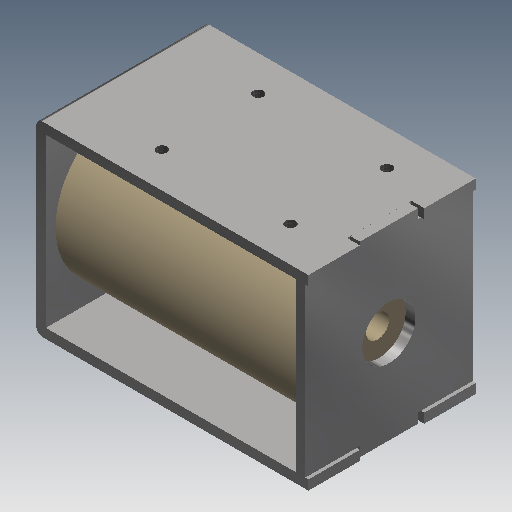
# Autodesk Inventor part: JF_0837B_Linear solenoid Pull 15N 12v1A Frame
Saved by Autodesk Inventor 2018.3 (Build 223284000, 284)
## iProperties
Manager: GURSKY
Company: ltd "MRF-ENGINEERING"
Created: 2017-09-28
Part Number: JF_0837B_Linear solenoid Pull 15N 12v1A Frame
Project: 1706
Checked By: Гурский
Engr Approved By: ---
Material: Сталь нержавеющая, 440C
Catalog Web Link: http://mrfengineering.com.ua/
Vendor: ltd "MRF-ENGINEERING"
Document SubType Name: Листовой металл
Designer: Макс
Engineer: TIHONOV
Authority: GURSKY
Stock Number: 1706
Density: 7.75 g/cm^3
Sheet Metal Rule: Default_mm
Appearance: С умеренной полировкой
Заготовка: ЛИСТ ГОРЯЧЕКАТАННЫЙ 4,0х1500х6000
Материал: Ст. 3СП/ПС
Title: ---
Subject: Filling mashine
Author: Макс
Autodesk Inventor part; units mm, degrees
ref_plane "YZ Plane" through (0, 0, 0) normal (1, 0, 0) x (0, 1, 0)
ref_plane "XZ Plane" through (0, 0, 0) normal (0, 1, 0) x (-1, 0, 0)
ref_plane "XY Plane" through (0, 0, 0) normal (0, 0, 1) x (1, 0, 0)
sketch "Эскиз2" plane through (0, 0, 0) normal (0, 0, 1) x (1, 0, 0)
  line L0 (84.6, 29) -> (2, 29)
  line L1 (0, 27) -> (0, -27)
  line L2 (2, -29) -> (84.6, -29)
  line L3 (84.6, -26) -> (3, -26)
  line L4 (3, -26) -> (3, 26)
  line L5 (3, 26) -> (84.6, 26)
  line L6 (84.6, -29) -> (84.6, -26)
  line L7 (84.6, 26) -> (84.6, 29)
  arc A0 (0, -27) -> (2, -29) centre (2, -27) ccw
  arc A1 (2, 29) -> (0, 27) centre (2, 27) ccw
  point P0 (0, 0)
  point P1 (0, -29)
  point P2 (0, 29)
  point P3 (0, 0)
  dimension "d0" = 84.6
  dimension "d1" = 3
  dimension "d2" = 58
  dimension "d34" = 2
  constraints: 16 end point, 4 point on circle, 4 point on line, 4 tangent, 3 equal length, 2 centre point, 2 perpendicular, 1 coincident, 1 collinear, 1 equal radius, 1 horizontal, 1 midpoint, 1 vertical, 2 other
  measures "d0" distance between parallel lines of L6 L1
  measures "d1" distance between parallel lines of L3 L2
  measures "d2" distance of point (0, 29) point (0, -29)
  measures "d34" radius of A0
extrude "Выдавливание1" add sketch "Эскиз2" along normal mid plane 52
sketch "Эскиз3" plane through (0, 29, 26) normal (0, 1, 0) x (1, 0, 0)
  line L0 (84.6, 0) -> (84.6, 52) projected
  point P0 (0, 26)
  point P1 (68, 11)
  point P2 (28, 11)
  point P3 (28, 41)
  point P4 (68, 41)
  dimension "d5" = 40
  dimension "d6" = 16.6
  dimension "d7" = 30
  dimension "d8" = 15
  constraints: 2 horizontal alignment, 2 vertical alignment
  measures "d5" distance of point (68, 11) point (28, 11)
  measures "d6" distance from line of L0 point (68, 11)
  measures "d7" distance of point (68, 41) point (68, 11)
  measures "d8" vertical distance of point (0, 26) point (68, 41)
hole "Отверстие1" at (68, 29, 15) at (28, 29, 15) at (28, 29, -15) at (68, 29, -15) direction (0, -1, 0) diameter 3.242 depth 3 tip angle 118 thread size "M4x0.7" class "6H" standard "ISO Metric profile"
sketch "Эскиз4" plane through (0, -29, 26) normal (-1, 0, 0) x (0, 0, 1)
  circle A0 centre (-26, 29) radius 3
  point P0 (-26, 29)
  dimension "d16" = 6
  constraints: 1 centre point, 1 coincident
  measures "d16" diameter of A0
extrude "Выдавливание2" cut sketch "Эскиз4" against normal blind 4
sketch "Эскиз5" plane through (0, 29, 26) normal (0, 1, 0) x (1, 0, 0)
  line L0 (80.6, 36) -> (84.6, 36)
  line L1 (84.6, 36) -> (84.6, 16)
  line L2 (84.6, 16) -> (80.6, 16)
  line L3 (80.6, 16) -> (80.6, 36)
  line L4 (84.6, 0) -> (84.6, 52) projected
  point P0 (0, 26)
  point P1 (84.6, 26)
  dimension "d19" = 4
  dimension "d20" = 20
  constraints: 8 end point, 2 midpoint, 2 parallel, 1 horizontal, 1 perpendicular
  measures "d19" distance of L1.end L2.end
  measures "d20" distance of L0.end L1.end
extrude "Выдавливание3" cut sketch "Эскиз5" against normal through all
sketch "Эскиз6" plane through (80.6, -29, 10) normal (1, 0, 0) x (0, 0, -1)
  line L0 (36, 3) -> (36, 55)
  line L1 (36, 55) -> (19, 55)
  line L2 (19, 55) -> (19, 58)
  line L3 (36, 58) -> (-16, 58)
  line L4 (19, 58) -> (1, 58)
  line L5 (1, 58) -> (1, 55)
  line L6 (1, 55) -> (-16, 55)
  line L7 (-16, 56) -> (-16, 2)
  line L8 (-16, 55) -> (-16, 3)
  line L9 (-16, 3) -> (1, 3)
  line L10 (1, 3) -> (1, 0)
  line L11 (1, 0) -> (19, 0)
  line L12 (36, 0) -> (-16, 0)
  line L13 (19, 0) -> (19, 3)
  line L14 (36, 3) -> (19, 3)
  line L15 (36, 55) -> (36, 3)
  point P0 (10, 29)
  point P1 (10, 0)
  dimension "d23" = 18
  dimension "d24" = 18
  constraints: 32 end point, 11 point on line, 5 perpendicular, 1 collinear, 1 horizontal, 1 midpoint, 1 vertical, 1 vertical alignment
  measures "d23" distance between parallel lines of L10 L13
  measures "d24" distance between parallel lines of L5 L2
extrude "Выдавливание4" add sketch "Эскиз6" along normal blind 3 separate body
sketch "Эскиз7" plane through (83.6, -29, 10) normal (1, 0, 0) x (0, 0, -1)
  circle A0 centre (10, 29) radius 8.25
  point P0 (10, 29)
  dimension "d27" = 16.5
  constraints: 1 centre point, 1 coincident
  measures "d27" diameter of A0
extrude "Выдавливание5" cut sketch "Эскиз7" against normal blind 3 bodies 2
sketch "Эскиз8" plane through (0, 0, 0) normal (0, 0, 1) x (1, 0, 0)
  line L0 (3.5, -23.5) -> (80.1, -23.5)
  line L1 (80.1, -23.5) -> (80.1, -3.6097)
  line L2 (80.1, -3.6097) -> (3.5, -3.6097)
  line L3 (3.5, -3.6097) -> (3.5, -23.5)
  line L4 (0, 0) -> (96.507, 0)
  line L5 (3, -26) -> (3, 26) projected
  line L6 (80.6, -26) -> (80.6, 26) projected
  dimension "d30" = 47
  dimension "d31" = 0.5
  dimension "d32" = 0.5
  constraints: 10 end point, 2 horizontal, 2 parallel, 1 perpendicular
  measures "d30" diameter of L0 L4
  measures "d31" distance between parallel lines of L5 L3
  measures "d32" distance between parallel lines of L6 L1
revolve "Вращение1" add sketch "Эскиз8" angle 360 about axis through (0, 0, 0) along (1, 0, 0) separate body
equation "\"d8\" = 0.5 * d7"
equation "\"d32\" = d31"
equation "\"Радиус_гибки\" = Толщина"
equation "\"Ширина_просечки\" = Толщина"
equation "\"Глубина_просечки\" = 0.5 * Толщина"
equation "\"Размер_просечки\" = 4 * Толщина"
equation "\"Мин_остаток\" = 2 * Толщина"
equation "\"Радиус_перехода\" = Радиус_гибки"
equation "\"Радиус_Якоби\" = Радиус_гибки"
equation "\"Размер_зазора\" = Толщина"
equation "\"Толщина\" = 2"
